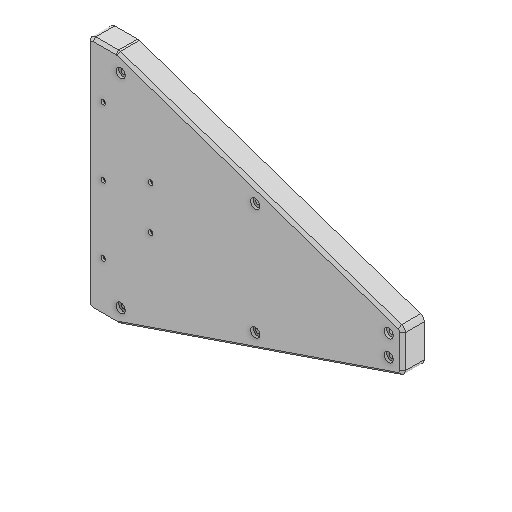
# Autodesk Inventor part: 3DP_PLA_Antenna_Case_Bottom
Saved by Autodesk Inventor 2026.1 (Build 301233000, 233)
## iProperties
Created: 2025-10-17
Part Number: 3DP_PLA_Antenna_Case_Bottom
Material: Generic
Document SubType Name: Modeling
Designer: User
Density: 1 g/cm^3
Appearance: Default
Author: User
Autodesk Inventor part; units mm, degrees
ref_plane "YZ Plane" through (0, 0, 0) normal (1, 0, 0) x (0, 1, 0)
ref_plane "XZ Plane" through (0, 0, 0) normal (0, 1, 0) x (-1, 0, 0)
ref_plane "XY Plane" through (0, 0, 0) normal (0, 0, 1) x (1, 0, 0)
sketch "Sketch1" plane through (0, 0, 0) normal (0, 0, 1) x (1, 0, 0)
  circle A0 centre (-98.0984, 74.6932) radius 1.75
  line L0 (-101.515, 79.4432) -> (103.485, 9.4432)
  circle A1 centre (1.4016, 40.6932) radius 1.75
  line L1 (103.485, 9.4432) -> (103.485, -10.5568)
  circle A2 centre (100.1516, -8.3068) radius 1.75
  line L2 (103.485, -10.5568) -> (-101.515, -80.5568)
  circle A3 centre (100.1516, 7.1932) radius 1.75
  circle A4 centre (1.4016, -41.8068) radius 1.75
  circle A5 centre (-98.0984, -75.8068) radius 1.75
  line L3 (-101.515, -80.5568) -> (-101.515, 79.4432)
  line L4 (106.5081, 11.581) -> (-101.5865, 82.6377)
  line L5 (-101.515, -83.7513) -> (106.5081, -12.719)
  line L6 (106.5081, -12.719) -> (106.5081, 11.581)
  line L7 (-101.5865, 82.6377) -> (-118.515, 82.6377)
  line L8 (-118.515, 82.6377) -> (-118.515, -83.7513)
  line L9 (-118.515, -83.7513) -> (-101.515, -83.7513)
  line L10 (-122.515, 86.6377) -> (-100.9224, 86.6377)
  line L11 (-100.9224, 86.6377) -> (110.5081, 14.4419)
  line L12 (110.5081, 14.4419) -> (110.5081, -15.5799)
  line L13 (110.5081, -15.5799) -> (-100.8509, -87.7513)
  line L14 (-100.8509, -87.7513) -> (-122.515, -87.7513)
  line L15 (-122.515, -87.7513) -> (-122.515, 86.6377)
  circle A6 centre (-98.0984, 74.6932) radius 6.5
  circle A7 centre (1.4016, 40.6932) radius 6.5
  circle A8 centre (100.1516, 7.1932) radius 6.5
  circle A9 centre (100.1516, -8.3068) radius 6.5
  circle A10 centre (1.4016, -41.8068) radius 6.5
  circle A11 centre (-98.0984, -75.8068) radius 6.5
  point P0 (-95.0293, -81.5366)
  point P1 (-97.022, -82.2171)
  point P2 (2.6291, -48.1898)
  point P3 (4.3345, -47.6075)
  point P4 (100.4087, -14.8017)
  point P5 (103.9207, -13.6025)
  point P6 (106.5081, -9.6655)
  point P7 (106.5081, -6.9481)
  point P8 (106.5081, 8.5519)
  point P9 (103.985, 12.4425)
  point P10 (100.3295, 13.6908)
  point P11 (106.5081, 5.8345)
  point P12 (4.4707, 46.423)
  point P13 (2.478, 47.1035)
  point P14 (-94.9118, 80.3585)
  point P15 (-97.1545, 81.1243)
  point P16 (-111, -50.5568)
  point P17 (-111, -0.5568)
  point P18 (-111, 49.4432)
  point P19 (-76, 15.4432)
  point P20 (-76, -16.5568)
  dimension "d0" = 205
  dimension "d1" = 160
  dimension "d2" = 20
  dimension "d3" = 71.147
  dimension "d4" = 3.4167
  dimension "d5" = 4.75
  dimension "d6" = 3.4167
  dimension "d7" = 4.75
  dimension "d8" = 38.75
  dimension "d9" = 72.25
  dimension "d10" = 102.9167
  dimension "d11" = 201.6667
  dimension "d12" = 201.6667
  dimension "d13" = 102.9167
  dimension "d14" = 38.75
  dimension "d15" = 72.25
  dimension "d16" = 3
  dimension "d18" = 17
  dimension "d19" = 4
  dimension "d24" = 13
  dimension "d25" = 13
  dimension "d26" = 13
  dimension "d27" = 13
  dimension "d28" = 13
  dimension "d29" = 13
  dimension "d33" = 3.5
  dimension "d34" = 3.5
  dimension "d35" = 3.5
  dimension "d36" = 3.5
  dimension "d37" = 3.5
  dimension "d38" = 3.5
  dimension "d64" = 17
  dimension "d65" = 100
  dimension "d66" = 166.3889
  dimension "d67" = 33.1945
  dimension "d68" = 50
  dimension "d76" = 16
  dimension "d77" = 16
  dimension "d78" = 35
  constraints: 32 end point, 12 centre point, 6 coincident, 4 perpendicular, 2 vertical alignment, 1 horizontal, 6 other
  measures "d0" distance between parallel lines of L1 L3
  measures "d1" distance of L2.end L0.start
  measures "d2" distance of L0.end L1.end
  measures "d3" angle of L3 L0
  measures "d4" distance from line of L3 A5.centre
  measures "d5" vertical distance of L2.end A5.centre
  measures "d6" distance from line of L3 A0.centre
  measures "d7" vertical distance of L0.start A0.centre
  measures "d8" vertical distance of A4.centre L2.end
  measures "d9" vertical distance of A2.centre L2.end
  measures "d10" distance from line of L3 A4.centre
  measures "d11" distance from line of L3 A2.centre
  measures "d12" distance from line of L3 A3.centre
  measures "d13" distance from line of L3 A1.centre
  measures "d14" vertical distance of A1.centre L0.start
  measures "d15" vertical distance of L0.start A3.centre
  measures "d16" distance between parallel lines of L0 L4
  measures "d18" distance between parallel lines of L3 L8
  measures "d19" distance between parallel lines of L7 L10
  measures "d24" diameter of A6
  measures "d25" diameter of A7
  measures "d26" diameter of A8
  measures "d27" diameter of A9
  measures "d28" diameter of A10
  measures "d29" diameter of A11
  measures "d33" diameter of A5
  measures "d34" diameter of A0
  measures "d35" diameter of A4
  measures "d36" diameter of A1
  measures "d37" diameter of A3
  measures "d38" diameter of A2
  measures "d64" distance of L8.end L5.start
  measures "d65" distance of point (-111, 49.443) point (-111, -50.557)
  measures "d66" distance between parallel lines of L7 L9
  measures "d67" distance from line of L9 point (-111, -50.557)
  measures "d68" distance of point (-111, -0.557) point (-111, -50.557)
  measures "d76" vertical distance of point (-111, -0.557) point (-76, 15.443)
  measures "d77" vertical distance of point (-111, -0.557) point (-76, -16.557)
  measures "d78" horizontal distance of point (-111, -0.557) point (-76, 15.443)
extrude "Extrusion1" add sketch "Sketch1" along normal blind 3 contours L3 A6 L4 L0 | L0 A6 L3 | A6 L4 A7 L0 | L0 A7 A8 L1 A9 L2 A10 A11 L3 A6 | L3 A11 L5 L9 L8 L7 L4 A6 | A7 L4 L0 | L0 A7 | L4 A6 | A11 L2 L3 | L3 L2 A11 L5 | A7 L4 A8 L0 | A7 L4 | L5 A11 | A8 L4 L6 L1 L0 | L0 L1 A8 | L2 A10 L5 A11 | A8 L4 | A8 L6 A9 L1 | A10 L2 | L2 A10 L5 | L5 A10 | L4 L6 A8 | A9 L6 L5 L2 L1 | L1 L2 A9 | L6 A8 | L2 A9 L5 A10 | A9 L6 | L5 A9 | L6 L5 A9 | L10 L11 L12 L13 L14 L15
extrude "Extrusion2" add sketch "Sketch1" against normal blind 13 contours L4 A6 | A7 L4 | L5 A11 | A8 L4 | L5 A10 | L6 A8 | A9 L6 | L5 A9 | L10 L11 L12 L13 L14 L15
extrude "Extrusion3" add sketch "Sketch1" against normal blind 12.2 contours L3 A6 L4 L0 | L0 A6 L3 | A7 L4 L0 | L0 A7 | A11 L2 L3 | L3 L2 A11 L5 | A8 L4 L6 L1 L0 | L0 L1 A8 | A10 L2 | L2 A10 L5 | L4 L6 A8 | A9 L6 L5 L2 L1 | L1 L2 A9 | L6 L5 A9
fillet "Fillet1" radius 2 12 edges at (-95.0293, -81.5366, -6.1) (2.6291, -48.1898, -6.1) (4.3345, -47.6075, -6.1) (100.4087, -14.8017, -6.1) (106.5081, -6.9481, -6.1) (106.5081, 5.8345, -6.1) (100.3295, 13.6908, -6.1) (2.478, 47.1035, -6.1) (4.4707, 46.423, -6.1) (-94.9118, 80.3585, -6.1) (-97.1545, 81.1243, -6.1) (-97.022, -82.2171, -6.1)
sketch "Sketch2" plane through (-122.515, -87.7513, 3) normal (-1, 0, 0) x (0, 0, 1)
  line L0 (0, 0) -> (-16, 0) projected
  line L1 (0, 174.3889) -> (0, 0) projected
  line L2 (-16, 174.3889) -> (0, 174.3889) projected
  line L3 (-16, 0) -> (-16, 174.3889) projected
  circle A0 centre (-17.825, 87.1945) radius 3.15
  point P0 (-3, 87.7513)
  dimension "d39" = 174.3889
  dimension "d40" = 87.1945
  dimension "d41" = 1.825
  dimension "d42" = 6.3
  constraints: 1 centre point, 1 coincident
  measures "d39" distance of L0.end L2.start
  measures "d40" distance from line of L0 point (-17.825, 87.194)
  measures "d41" distance from line of L3 point (-17.825, 87.194)
  measures "d42" diameter of A0
extrude "Extrusion4" cut sketch "Sketch2" against normal blind 11.2 contours A0 L3 | L3 A0
fillet "Fillet2" radius 1.5 24 edges at (-2.0797, 47.5824, 0) (-0.6988, 34.5419, 0) (8.3695, 44.0144, 0) (52.7579, 29.9347, 0) (96.4821, 13.9532, 0) (94.9036, 3.3581, 0) (105.4955, 1.6337, 0) (-91.1224, 77.9902, 0) (-100.36, 68.5993, 0) (-101.2403, 81.1736, 0) (-46.2728, 63.7501, 0) (-110.0507, 82.6377, 0) (-118.515, -0.5568, 0) (-110.015, -83.7513, 0) (52.765, -31.0703, 0) (-46.2653, -64.8855, 0) (-100.3713, -69.7172, 0) (-91.1305, -79.128, 0) (-2.0584, -48.7102, 0) (-0.6988, -35.6555, 0) (8.3613, -45.1523, 0) (96.5027, -15.0813, 0) (94.8976, -4.4799, 0) (105.4955, -2.7473, 0)
sketch "Sketch4" plane through (0, 0, 3) normal (0, 0, 1) x (1, 0, 0)
  line L0 (-122.515, -87.7513) -> (-100.8509, -87.7513) projected
  line L1 (-100.8509, -87.7513) -> (110.5081, -15.5799) projected
  line L2 (110.5081, -15.5799) -> (110.5081, 14.4419) projected
  line L3 (110.5081, 14.4419) -> (-100.9224, 86.6377) projected
  line L4 (-100.9224, 86.6377) -> (-122.515, 86.6377) projected
  line L5 (-122.515, 86.6377) -> (-122.515, -87.7513) projected
  circle A0 centre (-98.0984, 74.6932) radius 1.75 projected
  circle A1 centre (1.4016, 40.6932) radius 1.75 projected
  circle A2 centre (-98.0984, -75.8068) radius 1.75 projected
  circle A3 centre (1.4016, -41.8068) radius 1.75 projected
  circle A4 centre (100.1516, -8.3068) radius 1.75 projected
  circle A5 centre (100.1516, 7.1932) radius 1.75 projected
  circle A6 centre (-98.0984, 74.6932) radius 3.5
  circle A7 centre (1.4016, 40.6932) radius 3.5
  arc A8 (100.3295, 13.6908) -> (106.5081, 5.8345) centre (100.1516, 7.1932) ccw projected
  circle A9 centre (100.1516, 7.1932) radius 3.5
  circle A10 centre (100.1516, -8.3068) radius 3.5
  circle A11 centre (1.4016, -41.8068) radius 3.5
  circle A12 centre (-98.0984, -75.8068) radius 3.5
  point P0 (0, 0)
  point P1 (103.483, 1.6118)
  point P2 (95.8459, 12.0625)
  dimension "d52" = 7
  dimension "d53" = 7
  dimension "d54" = 7
  dimension "d55" = 7
  dimension "d56" = 7
  dimension "d57" = 7
  constraints: 6 centre point, 6 coincident
  measures "d52" diameter of A6
  measures "d53" diameter of A7
  measures "d54" diameter of A9
  measures "d55" diameter of A10
  measures "d56" diameter of A11
  measures "d57" diameter of A12
extrude "Extrusion5" cut sketch "Sketch4" against normal blind 2 contours A0 | A1 | A2 | A3 | A4 | A5 | A6 | A7 | A9 | A10 | A11 | A12
fillet "Fillet3" radius 4 10 edges at (-100.8509, -87.7513, -5) (110.5081, -15.5799, -5) (110.5081, 14.4419, -5) (-100.9224, 86.6377, -5) (-122.515, -87.7513, -5) (-122.515, 86.6377, -5) (-118.0757, 82.1983, -0.4393) (-118.515, 82.6377, -7.25) (-118.0757, -83.3119, -0.4393) (-118.515, -83.7513, -7.25)
chamfer "Chamfer1" distance 2 angle 45 12 edges at (3.7534, 50.8947, 3) (-100.9313, 86.5836, 3) (-110.0507, 86.6377, 3) (-121.3435, 85.4661, 3) (-122.515, -0.5568, 3) (-121.3435, -86.5797, 3) (-110.015, -87.7513, 3) (-100.8599, -87.6973, 3) (3.7891, -52.0205, 3) (109.7615, -15.046, 3) (110.5081, -0.569, 3) (109.7615, 13.908, 3)
hole "Hole1" at (-111, -50.5568, 0) at (-111, -0.5568, 0) at (-111, 49.4432, 0) at (-76, 15.4432, 0) at (-76, -16.5568, 0) direction (0, 0, 1) diameter 3.5 end through all
sketch "Sketch5" plane through (0, 0, 0) normal (0, 0, -1) x (-1, 0, 0)
  circle A0 centre (76, -16.5568) radius 1.75 projected
  circle A1 centre (76, 15.4432) radius 1.75 projected
  circle A2 centre (111, 49.4432) radius 1.75 projected
  circle A3 centre (111, -0.5568) radius 1.75 projected
  circle A4 centre (111, -50.5568) radius 1.75 projected
  arc A5 (114.515, -82.2513) -> (117.015, -79.7513) centre (114.515, -79.7513) ccw projected
  line L0 (117.015, 78.6377) -> (117.015, -79.7513) projected
  arc A6 (117.015, 78.6377) -> (114.515, 81.1377) centre (114.515, 78.6377) ccw projected
  line L1 (102.8518, 81.1377) -> (114.515, 81.1377) projected
  arc A7 (102.8518, 81.1377) -> (102.9158, 81.0801) centre (103.2168, 81.4793) ccw projected
  arc A8 (90.2805, 76.3908) -> (102.9158, 81.0801) centre (98.0984, 74.6932) ccw projected
  arc A9 (90.2805, 76.3908) -> (89.6304, 76.9701) centre (89.7919, 76.4969) ccw projected
  line L2 (3.8846, 47.691) -> (89.6304, 76.9701) projected
  arc A10 (3.8846, 47.691) -> (3.7257, 46.834) centre (4.0462, 47.2178) ccw projected
  arc A11 (-9.214, 42.4156) -> (3.7257, 46.834) centre (-1.4016, 40.6932) ccw projected
  arc A12 (-9.214, 42.4156) -> (-9.8639, 42.9964) centre (-9.7023, 42.5232) ccw projected
  line L3 (-94.6826, 14.0339) -> (-9.8639, 42.9964) projected
  arc A13 (-94.6826, 14.0339) -> (-94.8522, 13.1862) centre (-94.521, 13.5608) ccw projected
  arc A14 (-98.1673, -0.5568) -> (-94.8522, 13.1862) centre (-100.1516, 7.1932) ccw projected
  arc A15 (-94.871, -14.3164) -> (-98.1673, -0.5568) centre (-100.1516, -8.3068) ccw projected
  arc A16 (-94.871, -14.3164) -> (-94.7025, -15.1651) centre (-94.5409, -14.6919) ccw projected
  line L4 (-9.858, -44.1364) -> (-94.7025, -15.1651) projected
  arc A17 (-9.858, -44.1364) -> (-9.2085, -43.554) centre (-9.6964, -43.6632) ccw projected
  arc A18 (3.7062, -47.9639) -> (-9.2085, -43.554) centre (-1.4016, -41.8068) ccw projected
  arc A19 (3.7062, -47.9639) -> (3.8638, -48.8219) centre (4.0254, -48.3488) ccw projected
  line L5 (89.6361, -78.11) -> (3.8638, -48.8219) projected
  arc A20 (89.6361, -78.11) -> (90.286, -77.5292) centre (89.7977, -77.6368) ccw projected
  arc A21 (102.8715, -82.2268) -> (90.286, -77.5292) centre (98.0984, -75.8068) ccw projected
  arc A22 (102.8715, -82.2268) -> (102.8412, -82.2513) centre (103.1699, -82.6281) ccw projected
  line L6 (114.515, -82.2513) -> (102.8412, -82.2513) projected
  line L7 (109.389, 46.5405) -> (107.6807, 49.3871)
  line L8 (107.6807, 49.3871) -> (109.2917, 52.2897)
  line L9 (109.2917, 52.2897) -> (112.611, 52.3458)
  line L10 (112.611, 52.3458) -> (114.3193, 49.4993)
  line L11 (114.3193, 49.4993) -> (112.7083, 46.5967)
  line L12 (112.7083, 46.5967) -> (109.389, 46.5405)
  line L13 (74.3401, 12.5682) -> (72.6802, 15.4432)
  line L14 (72.6802, 15.4432) -> (74.3401, 18.3182)
  line L15 (74.3401, 18.3182) -> (77.6599, 18.3182)
  line L16 (77.6599, 18.3182) -> (79.3198, 15.4432)
  line L17 (79.3198, 15.4432) -> (77.6599, 12.5682)
  line L18 (77.6599, 12.5682) -> (74.3401, 12.5682)
  line L19 (109.3401, -3.4318) -> (107.6802, -0.5568)
  line L20 (107.6802, -0.5568) -> (109.3401, 2.3182)
  line L21 (109.3401, 2.3182) -> (112.6599, 2.3182)
  line L22 (112.6599, 2.3182) -> (114.3198, -0.5568)
  line L23 (114.3198, -0.5568) -> (112.6599, -3.4318)
  line L24 (112.6599, -3.4318) -> (109.3401, -3.4318)
  line L25 (74.4019, -19.4666) -> (72.681, -16.6277)
  line L26 (72.681, -16.6277) -> (74.2791, -13.7179)
  line L27 (74.2791, -13.7179) -> (77.5981, -13.647)
  line L28 (77.5981, -13.647) -> (79.319, -16.4859)
  line L29 (79.319, -16.4859) -> (77.7209, -19.3957)
  line L30 (77.7209, -19.3957) -> (74.4019, -19.4666)
  line L31 (109.3401, -53.4318) -> (107.6802, -50.5568)
  line L32 (107.6802, -50.5568) -> (109.3401, -47.6818)
  line L33 (109.3401, -47.6818) -> (112.6599, -47.6818)
  line L34 (112.6599, -47.6818) -> (114.3198, -50.5568)
  line L35 (114.3198, -50.5568) -> (112.6599, -53.4318)
  line L36 (112.6599, -53.4318) -> (109.3401, -53.4318)
  point P0 (0, 0)
  point P1 (76.0614, -19.4311)
  dimension "d79" = 5.75
  dimension "d80" = 5.75
  dimension "d81" = 5.75
  dimension "d82" = 5.75
  dimension "d83" = 5.75
  constraints: 60 end point, 5 coincident, 1 midpoint, 1 point on line, 65 other
  measures "d79" distance between parallel lines of L33 L36
  measures "d80" distance between parallel lines of L30 L27
  measures "d81" distance between parallel lines of L24 L21
  measures "d82" distance between parallel lines of L15 L18
  measures "d83" distance between parallel lines of L9 L12
extrude "Extrusion6" cut sketch "Sketch5" against normal blind 1.5 contours L7 L8 L9 L10 L11 L12 | L13 L14 L15 L16 L17 L18 | L19 L20 L21 L22 L23 L24 | L25 L26 L27 L28 L29 L30 | L31 L32 L33 L34 L35 L36
sketch "Sketch6" plane through (-118.515, -0.5568, -14.825) normal (1, 0, 0) x (0, 0, -1)
  arc A0 (-1.825, 2.5675) -> (-1.825, -2.5675) centre (0, 0) ccw projected
  line L0 (-2.4537, -4.25) -> (-4.9075, 0)
  line L1 (-4.9075, 0) -> (-2.4537, 4.25)
  line L2 (-2.4537, 4.25) -> (2.4537, 4.25)
  line L3 (2.4537, 4.25) -> (4.9075, 0)
  line L4 (4.9075, 0) -> (2.4537, -4.25)
  line L5 (2.4537, -4.25) -> (-2.4537, -4.25)
  point P0 (-14.825, 0.5568)
  dimension "d86" = 8.5
  constraints: 12 end point, 1 coincident, 13 other
  measures "d86" distance between parallel lines of L2 L5
extrude "Extrusion7" cut sketch "Sketch6" against normal blind 1
equation "\"d25\" = d24"
equation "\"d26\" = d24"
equation "\"d27\" = d24"
equation "\"d28\" = d24"
equation "\"d29\" = d24"
equation "\"d67\" = -0.5 * d65 + 0.5 * d66"
equation "\"d68\" = 0.5 * d65"
equation "\"d77\" = d76"
equation "\"d40\" = 0.5 * d39"
body "Solid1"
